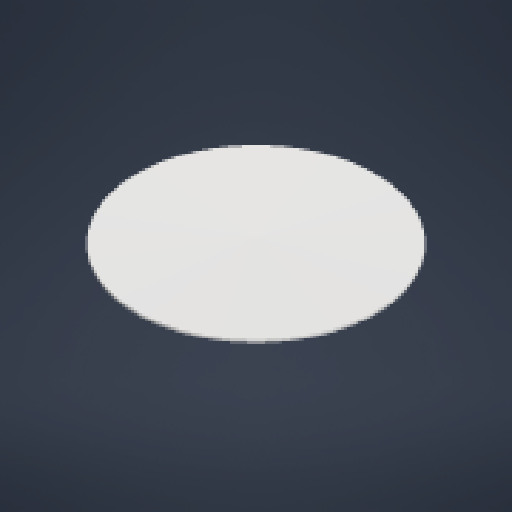
# Autodesk Inventor part: centrer centrifugal spinner
Saved by Autodesk Inventor 2026.1 (Build 301233000, 233)
## iProperties
Created: 2026-03-26
Part Number: centrer centrifugal spinner
Material: Generic
Document SubType Name: Modeling
Designer: sniel
Density: 1 g/cm^3
Appearance: Default
Author: sniel
Autodesk Inventor part; units mm, degrees
ref_plane "YZ Plane" through (0, 0, 0) normal (1, 0, 0) x (0, 1, 0)
ref_plane "XZ Plane" through (0, 0, 0) normal (0, 1, 0) x (-1, 0, 0)
ref_plane "XY Plane" through (0, 0, 0) normal (0, 0, 1) x (1, 0, 0)
sketch "Sketch1" plane through (0, 0, 0) normal (0, 0, 1) x (1, 0, 0)
  line L0 (0, 0) -> (98, 0)
  line L1 (0, 0) -> (-98, 0)
  line L2 (0, 0) -> (0, 5)
  line L3 (-98, 0) -> (-98, 2)
  line L4 (-98, 2) -> (0, 5)
  line L5 (0, 5) -> (0, 3)
  line L6 (0, 3) -> (-98, 0)
  line L7 (0, 3) -> (0, 0)
  line L8 (0, 0) -> (-5, 0)
  line L9 (-5, 0) -> (-5.0871, 2.8443)
  line L10 (-5, 0) -> (-5, -20)
  line L11 (-5, -20) -> (0, -20)
  line L12 (0, -20) -> (0, 0)
  line L13 (0, -25) -> (0, 10) projected
  dimension "d0" = 98
  dimension "d1" = 98
  dimension "d2" = 5
  dimension "d3" = 2
  dimension "d4" = 2
  dimension "d5" = 5
  dimension "d6" = 20
  constraints: 26 end point, 5 perpendicular, 4 point on line, 2 horizontal, 2 vertical
  measures "d0" distance of L0.start L0.end
  measures "d1" distance of L0.start L1.end
  measures "d2" distance of L0.start L2.end
  measures "d3" distance of L1.end L3.end
  measures "d4" distance of L2.end L5.end
  measures "d5" distance of L0.start L8.end
  measures "d6" distance of L8.end L10.end
revolve "Revolution1" add sketch "Sketch1" angle 360 about axis through (0, -10, 0) along (0, 1, 0) contours L12 L11 L10 L1 | L1 L9 L6 L2 | L6 L3 L4 L2
body "Solid1"
